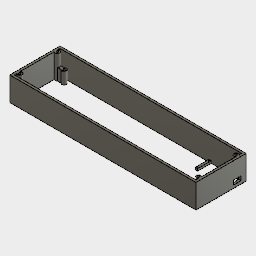
Project M404 v11 (Autodesk Fusion 360 design; units mm, degrees)
Autodesk Fusion 360 part; units mm, degrees
sketch "BoardFootprint" plane through (0, 0, 0) normal (0, 1, 0) x (1, 0, 0)
  line L0 (115, -30) -> (-115, -30)
  line L1 (-115, -30) -> (-115, 30)
  line L2 (-115, 30) -> (115, 30)
  line L3 (115, 30) -> (115, -30)
  line L4 (115, -30) -> (-115, 30) construction
  line L5 (-115, -30) -> (115, 30) construction
  circle A0 centre (-110, -25) radius 3
  circle A1 centre (-110, -25) radius 1.4
  circle A2 centre (110, -25) radius 3
  circle A3 centre (110, -25) radius 1.4
  circle A4 centre (-110, 25) radius 3
  circle A5 centre (-110, 25) radius 1.4
  circle A6 centre (110.2395, -0.0011) radius 3
  circle A7 centre (110.2395, -0.0011) radius 1.4
  dimension "d8" = 230
  dimension "d9" = 60
  dimension "d12" = 6
  dimension "d13" = 2.8
  dimension "d14" = 5
  dimension "d15" = 5
  dimension "d16" = 6
  dimension "d17" = 2.8
  dimension "d18" = 220
  dimension "d19" = 6
  dimension "d20" = 2.8
  dimension "d21" = 50
  dimension "d22" = 6
  dimension "d23" = 2.8
  dimension "d24" = 25
  dimension "d111" = 5
  dimension "d112" = 5
  measures "d8" distance of L0.start L0.end
  measures "d9" distance of L0.end L1.end
  measures "d12" diameter of A0
  measures "d13" diameter of A1
  measures "d14" distance of L0 A0.centre
  measures "d15" distance of L1 A0.centre
  measures "d16" diameter of A2
  measures "d17" diameter of A3
  measures "d18" distance of A0.centre A2.centre
  measures "d19" diameter of A4
  measures "d20" diameter of A5
  measures "d21" distance of A0.centre A4.centre
  measures "d22" diameter of A6
  measures "d23" diameter of A7
  measures "d24" distance of A2.centre A6.centre
  measures "d111" distance of L1 A4.centre
  measures "d112" distance of L0 A2.centre
sketch "Frame" plane through (0, 0, 0) normal (0, 1, 0) x (1, 0, 0)
  circle A0 centre (-119, -25) radius 3
  circle A1 centre (-119, -25) radius 1.4
  circle A2 centre (-119, 25) radius 3
  circle A3 centre (-119, 25) radius 1.4
  line L0 (115, -30) -> (-115, -30)
  circle A4 centre (119, -25) radius 3
  circle A5 centre (119, -25) radius 1.4
  circle A6 centre (119, 25) radius 3
  circle A7 centre (119, 25) radius 1.4
  line L1 (-122, 28) -> (-116, 28) construction
  line L2 (-115, 30) -> (115, 30)
  line L3 (-124, 33.5) -> (124, 33.5)
  line L4 (124, 33.5) -> (124, -33.5)
  line L5 (124, -33.5) -> (-124, -33.5)
  line L6 (-124, -33.5) -> (-124, 33.5)
  line L7 (-122, 27.5) -> (-122, 22.5) construction
  line L8 (122, -22.5) -> (122, -27.5) construction
  line L9 (-121, 30.5) -> (121, 30.5)
  line L10 (121, 30.5) -> (121, -30.5)
  line L11 (121, -30.5) -> (-121, -30.5)
  line L12 (-121, -30.5) -> (-121, 30.5)
  point P0 (-110, -25)
  point P1 (-110, 25)
  point P2 (110, -25)
  dimension "d26" = 6
  dimension "d27" = 2.8
  dimension "d28" = 6
  dimension "d29" = 2.8
  dimension "d30" = 50
  dimension "d31" = 9
  dimension "d33" = 9
  dimension "d34" = 5
  dimension "d35" = 6
  dimension "d36" = 2.8
  dimension "d37" = 5
  dimension "d39" = 6
  dimension "d40" = 2.8
  dimension "d41" = 50
  dimension "d44" = 2
  dimension "d52" = 0.5
  dimension "d53" = 3
  dimension "d54" = 3
  dimension "d56" = 0.5
  dimension "d57" = 2
  dimension "d58" = 3
  dimension "d59" = 3
  dimension "d116" = 248
  measures "d26" diameter of A0
  measures "d27" diameter of A1
  measures "d28" diameter of A2
  measures "d29" diameter of A3
  measures "d30" distance of A0.centre A2.centre
  measures "d31" distance of A0.centre P0
  measures "d33" distance of A2.centre P1
  measures "d34" distance of A0.centre L0
  measures "d35" diameter of A4
  measures "d36" diameter of A5
  measures "d37" distance of L0 A4.centre
  measures "d39" diameter of A6
  measures "d40" diameter of A7
  measures "d41" distance of A6.centre P2
  measures "d44" distance of L6 L7
  measures "d52" distance of L2 L9
  measures "d53" distance of L3 L9
  measures "d54" distance of L6 L12
  measures "d56" distance of L0 L11
  measures "d57" distance of L4 L8
  measures "d58" distance of L5 L11
  measures "d59" distance of L4 L10
  measures "d116" distance of L4 L6
sketch "Interconnects" plane through (0, 0, 0) normal (0, 1, 0) x (1, 0, 0)
  line L0 (-117.6, 27) -> (-111.4, 27)
  line L1 (-111.4, 27) -> (-111.4, 23)
  line L2 (-111.4, 23) -> (-117.6, 23)
  line L3 (-117.6, 23) -> (-117.6, 27)
  circle A0 centre (-119, 25) radius 1.4
  circle A1 centre (-119, 25) radius 1.4
  circle A2 centre (-119, 25) radius 1.4
  circle A3 centre (-110, 25) radius 1.4
  line L4 (-117.6, -23) -> (-111.4, -23)
  line L5 (-111.4, -23) -> (-111.4, -27)
  line L6 (-111.4, -27) -> (-117.6, -27)
  line L7 (-117.6, -27) -> (-117.6, -23)
  line L8 (-120, -23) -> (-109, -23) construction
  line L9 (-120, -27) -> (-109, -27) construction
  circle A4 centre (-119, -25) radius 3
  circle A5 centre (-119, -25) radius 3
  circle A6 centre (-119, -25) radius 1.4
  circle A7 centre (-110, -25) radius 1.4
  circle A8 centre (-119, -25) radius 1.4
  circle A9 centre (-119, -25) radius 3
  circle A10 centre (-119, -25) radius 1.4
  line L10 (-119, 25) -> (-110, 25) construction
  line L11 (-119, -25) -> (-110, -25) construction
  line L12 (110, -25) -> (119, -25) construction
  line L13 (111.4, -23) -> (117.6, -23)
  line L14 (117.6, -23) -> (117.6, -27)
  line L15 (117.6, -27) -> (111.4, -27)
  line L16 (111.4, -27) -> (111.4, -23)
  circle A11 centre (119, -25) radius 1.4
  circle A12 centre (110, -25) radius 1.4
  line L17 (108.8395, 1.9989) -> (121, 1.9989)
  line L18 (121, 1.9989) -> (121, -2.0011)
  line L19 (121, -2.0011) -> (108.8395, -2.0011)
  line L20 (108.8395, -2.0011) -> (108.8395, 1.9989)
  line L21 (110.2395, -0.0011) -> (122, -0.0011) construction
  circle A13 centre (110.2395, -0.0011) radius 1.4
  line L22 (121, 30.5) -> (121, -30.5)
  point P0 (110, -25)
  point P1 (119, -25)
  point P2 (110.2395, -0.0011)
  dimension "d60" = 4
  dimension "d61" = 4
  dimension "d62" = 4
  dimension "d64" = 4
  measures "d60" distance of L0.end L1.end
  measures "d61" distance of L4.end L5.end
  measures "d62" distance of L13.start L15.end
  measures "d64" distance of L17.start L19.end
extrude "Extrude1" add sketch "BoardFootprint" sketch "Interconnects" against normal blind 16 contours A0 | A2 | A4 | A6 of sketch 2 contours L0 L1 L2 L3 | L4 L6 L7 A4 A5 A9 | L4 L5 L6 A4 A5 A9 | L13 L14 L15 L16 | A13 | L17 L18 L19 L20 L22 picked at (-117.2323, -26.2179) makes body 1 at (-108.8955, -10.6667, 27.7893) makes body 2 at (112.2704, -10.6667, 2.2092) makes body 3 at (-108.8955, -10.6667, -22.2107) makes body 4 at (112.0309, -10.6667, 27.2081)
extrude "Extrude2" add sketch "Frame" against normal blind 16 contours A0 L12 | A0 L12 | A2 L12 | A2 L12 | A4 L10 | A4 L10 | A6 L10 | A6 L10 | L3 L4 L5 L6 bodies 1 2 3 4
extrude "Extrude3" add sketch "Frame" along normal blind 16 contours A0 L12 | A0 L12 | A2 L12 | A2 L12 | A4 L10 | A4 L10 | A6 L10 | A6 L10 | L3 L4 L5 L6 bodies 1
extrude "Extrude4" cut sketch "Frame" against normal blind 18 contours A6 L10 picked at (120.8, 25) bodies 1
sketch "NanoMountR" plane through (121, 0, 0) normal (-1, 0, 0) x (0, 0, 1)
  line L0 (-1.9989, -16) -> (-1.9989, 0)
  line L1 (-1.9989, 0) -> (2.0011, 0)
  line L2 (2.0011, 0) -> (2.0011, -16)
  line L3 (2.0011, -16) -> (22.7639, -16)
  line L4 (22.7639, -16) -> (22.7639, 16)
  line L5 (22.7639, 16) -> (-22.7639, 16)
  line L6 (-22.7639, 16) -> (-22.7639, 0)
  line L7 (-22.7639, 0) -> (-27.2361, 0)
  line L8 (-27.2361, 0) -> (-27.2361, 16)
  line L9 (-27.2361, 16) -> (-30.5, 16)
  line L10 (-30.5, 16) -> (-30.5, -16)
  line L11 (-30.5, -16) -> (-1.9989, -16)
  line L12 (-30.5, -16) -> (-27.5, -16)
  line L13 (-27.5, -16) -> (-27.5, -13)
  line L14 (-27.5, -13) -> (-30.5, -13)
  line L15 (-30.5, -13) -> (-30.5, -16)
  line L16 (-15.5, -16) -> (-12.5, -16)
  line L17 (-15.5, -13) -> (-15.5, -16)
  line L18 (-12.5, -16) -> (-12.5, -13)
  line L19 (-12.5, -13) -> (-15.5, -13)
  point P0 (-15.5, -16)
  dimension "d73" = 3
  dimension "d74" = 3
  dimension "d75" = 3
  dimension "d76" = 3
  dimension "d77" = 12
  measures "d73" distance of L13.end L14.end
  measures "d74" distance of L12.end L13.end
  measures "d75" distance of L17.start L18.end
  measures "d76" distance of L16.end L18.end
  measures "d77" distance of L13 L17
extrude "Extrude5" add sketch "NanoMountR" along normal blind 3.2 contours L11 L16 L17 L18 L19 | L10 L11 L12 L13 L14 L15 bodies 1
sketch "NanoMountL" plane through (0, -13, 0) normal (0, 1, 0) x (-1, 0, 0)
  line L0 (-121, -27.5) -> (-121, -30.5)
  line L1 (-121, -30.5) -> (-117.8, -30.5)
  line L2 (-117.8, -30.5) -> (-117.8, -27.5)
  line L3 (-117.8, -27.5) -> (-121, -27.5)
  circle A0 centre (-119.4, -29) radius 0.5
  circle A1 centre (-119.4, -14) radius 0.5
  line L4 (-77, -30.5) -> (-80.2, -30.5)
  line L5 (-80.2, -30.5) -> (-80.2, -12.5)
  line L6 (-80.2, -12.5) -> (-77, -12.5)
  line L7 (-77, -12.5) -> (-77, -30.5)
  circle A2 centre (-78.6, -29) radius 0.5
  circle A3 centre (-78.6, -14) radius 0.5
  line L8 (121, -30.5) -> (-121, -30.5)
  line L9 (-121, -22.7639) -> (-121, 22.7639)
  line L10 (-117.8, -12.5) -> (-117.8, -15.5)
  line L11 (-121, -12.5) -> (-117.8, -12.5)
  point P0 (-121, -12.5)
  dimension "d80" = 1
  dimension "d81" = 1
  dimension "d82" = 15
  dimension "d83" = 1
  dimension "d84" = 1
  dimension "d85" = 15
  dimension "d98" = 1.5
  dimension "d99" = 1.5
  dimension "d100" = 40.8
  dimension "d101" = 1.6
  dimension "d102" = 37.6
  measures "d80" diameter of A0
  measures "d81" diameter of A1
  measures "d82" distance of A0.centre A1.centre
  measures "d83" diameter of A2
  measures "d84" diameter of A3
  measures "d85" distance of A3.centre A2.centre
  measures "d98" distance of L4 A2.centre
  measures "d99" distance of A0.centre L8
  measures "d100" distance of A1.centre A3.centre
  measures "d101" distance of A1.centre L9
  measures "d102" distance of L5 L10
extrude "Extrude6" add sketch "NanoMountL" against normal blind 3 contours L4 L5 L6 L7 L8 bodies 1
extrude "Extrude7" cut sketch "NanoMountL" against normal blind 3 contours A0 | A1 bodies 1
sketch "USBPort" plane through (121, 0, 0) normal (-1, 0, 0) x (0, 0, 1)
  line L0 (-15.5, -16) -> (-15.5, -13)
  line L1 (-15.5, -13) -> (-12.5, -13)
  line L2 (-12.5, -13) -> (-12.5, -16)
  line L3 (-12.5, -16) -> (-1.9989, -16)
  line L4 (-1.9989, -16) -> (-1.9989, 0)
  line L5 (-1.9989, 0) -> (2.0011, 0)
  line L6 (2.0011, 0) -> (2.0011, -16)
  line L7 (2.0011, -16) -> (22.7639, -16)
  line L8 (22.7639, -16) -> (22.7639, 16)
  line L9 (22.7639, 16) -> (-22.7639, 16)
  line L10 (-22.7639, 16) -> (-22.7639, 0)
  line L11 (-22.7639, 0) -> (-27.2361, 0)
  line L12 (-27.2361, 0) -> (-27.2361, 16)
  line L13 (-27.2361, 16) -> (-30.5, 16)
  line L14 (-30.5, 16) -> (-30.5, -13)
  line L15 (-30.5, -13) -> (-27.5, -13)
  line L16 (-27.5, -13) -> (-27.5, -16)
  line L17 (-27.5, -16) -> (-15.5, -16)
  line L18 (-26.5, -6.5) -> (-16.5, -6.5)
  line L19 (-16.5, -6.5) -> (-16.5, -12)
  line L20 (-16.5, -12) -> (-26.5, -12)
  line L21 (-26.5, -12) -> (-26.5, -6.5)
  line L22 (-12.5, -13) -> (-30.5, -13)
  line L23 (-21.5, -13) -> (-21.5, -5.5) construction
  dimension "d93" = 10
  dimension "d94" = 5.5
  dimension "d95" = 1
  measures "d93" distance of L18.start L18.end
  measures "d94" distance of L18.start L20.end
  measures "d95" distance of L20 L22
extrude "Extrude8" cut sketch "USBPort" against normal blind 4 contours L18 L19 L20 L21 bodies 1
sketch "Facia" plane through (0, 16, 0) normal (0, 1, 0) x (-1, 0, 0)
  circle A0 centre (-119, 25) radius 1.4
  circle A1 centre (119, 25) radius 1.4
  line L0 (-121, 30.5) -> (121, 30.5)
  line L1 (121, 30.5) -> (121, 27.2361)
  arc A2 (121, 27.2361) -> (121, 22.7639) centre (119, 25) ccw
  line L2 (121, 22.7639) -> (121, -22.7639)
  arc A3 (121, -22.7639) -> (121, -27.2361) centre (119, -25) ccw
  line L3 (121, -27.2361) -> (121, -30.5)
  line L4 (121, -30.5) -> (-121, -30.5)
  line L5 (-121, -30.5) -> (-121, -27.2361)
  arc A4 (-121, -27.2361) -> (-121, -22.7639) centre (-119, -25) ccw
  line L6 (-121, -22.7639) -> (-121, 22.7639)
  arc A5 (-121, 22.7639) -> (-121, 27.2361) centre (-119, 25) ccw
  line L7 (-121, 27.2361) -> (-121, 30.5)
  circle A6 centre (-119, -25) radius 1.4
  circle A7 centre (119, -25) radius 1.4
  line L8 (124, 33.5) -> (-124, 33.5)
  line L9 (-124, 33.5) -> (-124, -33.5)
  line L10 (-124, -33.5) -> (124, -33.5)
  line L11 (124, -33.5) -> (124, 33.5)
  line L12 (124.125, -33.625) -> (-124.125, -33.625)
  line L13 (-124.125, -33.625) -> (-124.125, 33.625)
  line L14 (-124.125, 33.625) -> (124.125, 33.625)
  line L15 (124.125, 33.625) -> (124.125, -33.625)
  line L16 (124, 33.5) -> (124, -33.5)
  line L17 (-124, -33.5) -> (-124, 33.5)
  line L18 (-124, 33.5) -> (124, 33.5)
  circle A8 centre (-119, 25) radius 1.9
  circle A9 centre (-119, -25) radius 1.9
  circle A10 centre (119, -25) radius 1.9
  circle A11 centre (119, 25) radius 1.9
  dimension "d103" = 0.125
  dimension "d104" = 0.125
  dimension "d105" = 0.125
  dimension "d106" = 0.125
  dimension "d107" = 3.8
  dimension "d108" = 3.8
  dimension "d109" = 3.8
  dimension "d110" = 3.8
  measures "d103" distance of L10 L12
  measures "d104" distance of L15 L16
  measures "d105" distance of L13 L17
  measures "d106" distance of L14 L18
  measures "d107" diameter of A8
  measures "d108" diameter of A9
  measures "d109" diameter of A10
  measures "d110" diameter of A11
extrude "Extrude9" cut sketch "BoardFootprint" against normal blind 61 contours A3 | A7 bodies 1
equation "VFDBoardWidth = 230 mm"
equation "VFDBoardHeight = 60 mm"
equation "LLPostVerticalOffset = 5 mm"
equation "LLPostHorizontalOffset = 5 mm"
equation "PostVerticalOffset1 = 50 mm"
equation "PostVerticalOffset2 = 25 mm"
equation "PostHorizontalOffset = 220 mm"
equation "d8 = VFDBoardWidth"
equation "d9 = VFDBoardHeight"
equation "PostInnerDiameter = 2.8 mm"
equation "PostOuterDiameter = 6 mm"
equation "d12 = PostOuterDiameter"
equation "d13 = PostInnerDiameter"
equation "d14 = LLPostVerticalOffset"
equation "d15 = LLPostHorizontalOffset"
equation "d16 = PostOuterDiameter"
equation "d17 = PostInnerDiameter"
equation "d18 = PostHorizontalOffset"
equation "d19 = PostOuterDiameter"
equation "d20 = PostInnerDiameter"
equation "d21 = PostVerticalOffset1"
equation "d22 = PostOuterDiameter"
equation "d23 = PostInnerDiameter"
equation "d24 = PostVerticalOffset2"
equation "d26 = PostOuterDiameter"
equation "d27 = PostInnerDiameter"
equation "d28 = PostOuterDiameter"
equation "d29 = PostInnerDiameter"
equation "d30 = PostVerticalOffset1"
equation "d31 = FaciaPostHorizontalOffset"
equation "FaciaPostHorizontalOffset = 9 mm"
equation "d33 = FaciaPostHorizontalOffset"
equation "d34 = LLPostVerticalOffset"
equation "d35 = PostOuterDiameter"
equation "d36 = PostInnerDiameter"
equation "d37 = LLPostVerticalOffset"
equation "d39 = PostOuterDiameter"
equation "d40 = PostInnerDiameter"
equation "d41 = PostVerticalOffset1"
equation "d44 = FramePostOffset"
equation "FrameThickness = 3 mm"
equation "FramePostOffset = 2 mm"
equation "FrameInnerSlop = 0.5 mm"
equation "d52 = FrameInnerSlop"
equation "d53 = FrameThickness"
equation "d54 = FrameThickness"
equation "d56 = FrameInnerSlop"
equation "d57 = FramePostOffset"
equation "d58 = FrameThickness"
equation "d59 = FrameThickness"
equation "d61 = InterconnectThickness"
equation "d62 = InterconnectThickness"
equation "InterconnectThickness = 4 mm"
equation "d64 = InterconnectThickness"
equation "USBPortWidth = 10 mm"
equation "USBPortHeight = 5.5 mm"
equation "USBPortVerticalOffset = 1 mm"
equation "d93 = USBPortWidth"
equation "d94 = USBPortHeight"
equation "d95 = USBPortVerticalOffset"
equation "d107 = PostInnerDiameter + 1.0 mm"
equation "d108 = PostInnerDiameter + 1 mm"
equation "d109 = PostInnerDiameter + 1 mm"
equation "d110 = PostInnerDiameter + 1 mm"
